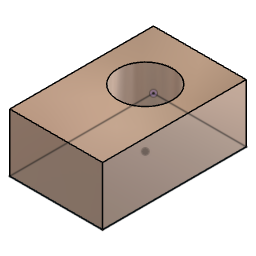
Lakeshore DT670 C0 clamp outline v2 (Autodesk Fusion 360 design; units mm, degrees)
Autodesk Fusion 360 part; units mm, degrees
note: some values were not read from the file. Set by a fixed rule: the direction of a hole.
sketch "Sketch1" plane through (0, 0, 0) normal (0, 1, 0) x (1, 0, 0)
  line L0 (0, 0) -> (5.1, 0)
  line L1 (5.1, 0) -> (5.1, -7.9)
  line L2 (5.1, -7.9) -> (0, -7.9)
  line L3 (0, -7.9) -> (0, 0)
  point P0 (2.55, -3)
  dimension "d1" = 5.1
  dimension "d2" = 7.9
  dimension "d5" = 2.55
  dimension "d6" = 3
  constraint horizontal L0
  constraint vertical L1
  constraint horizontal L2
  constraint vertical L3
  constraint coincident L0.start L3.end
  measures "d1" distance of L0.start L0.end
  measures "d2" distance of L0.start L2.end
  measures "d5" distance of L1 P0
  measures "d6" distance of L0 P0
extrude "Extrude1" add sketch "Sketch1" along normal blind 3.2
hole "Hole1" at (2.55, 0, 3) direction (0, 1, 0) diameter 3 depth 8 tip angle 118
equation "d5 = ( 5.1 / 2 ) * 1 mm"
